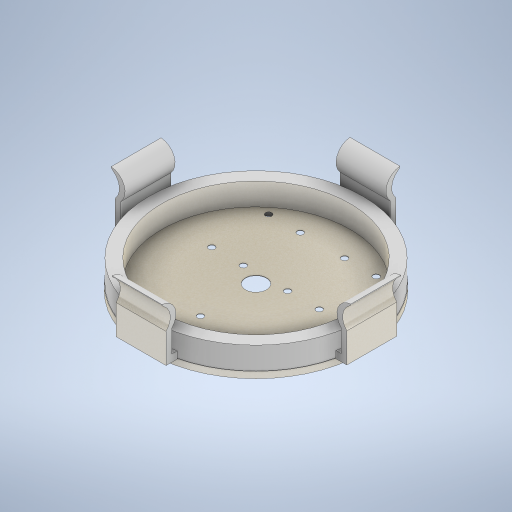
# Autodesk Inventor part: TapaContenedorTest
Saved by Autodesk Inventor 2024 (Build 280153000, 153)
## iProperties
Created: 2024-05-15
Part Number: TapaContenedorTest
Material: Genérico
Document SubType Name: Modeling
Designer: alexa
Density: 1 g/cm^3
Appearance: Valor por defecto
Author: alexa
Autodesk Inventor part; units mm, degrees
ref_plane "YZ Plane" through (0, 0, 0) normal (1, 0, 0) x (0, 1, 0)
ref_plane "XZ Plane" through (0, 0, 0) normal (0, 1, 0) x (-1, 0, 0)
ref_plane "XY Plane" through (0, 0, 0) normal (0, 0, 1) x (1, 0, 0)
sketch "Sketch1" plane through (0, 0, 0) normal (0, 1, 0) x (-1, 0, 0)
  circle A0 centre (0, 0) radius 50.9
  dimension "d0" = 101.8
  constraints: 1 centre point, 1 coincident
  measures "d0" diameter of A0
extrude "Extrusion1" add sketch "Sketch1" along normal blind 0.2
sketch "Sketch2" plane through (0, 0.2, 0) normal (0, 1, 0) x (1, 0, 0)
  circle A0 centre (0, 0) radius 50.675
  circle A1 centre (0, 0) radius 44.675
  dimension "d3" = 6
  dimension "d49" = 89.35
  constraints: 2 centre point, 1 coincident
  measures "d3" radial gap between concentric circles of A0 A1
  measures "d49" diameter of A1
extrude "Extrusion2" add sketch "Sketch2" along normal blind 10.6
sketch "Sketch3" plane through (0, 0, 0) normal (0, -1, 0) x (1, 0, 0)
  circle A0 centre (0, 0) radius 50.9 projected
  line L0 (-54.6995, -11.6386) -> (-54.6995, 12.0614)
  line L1 (-54.6995, -11.6386) -> (-49.5515, -11.6386)
  line L2 (-54.6995, 12.0614) -> (-49.4503, 12.0614)
  dimension "d8" = 23.7
  constraints: 6 end point, 2 point on circle, 1 horizontal, 1 parallel
  measures "d8" distance of L0.start L0.end
extrude "Extrusion3" add sketch "Sketch3" against normal blind 3.4 contours A0 L1 L0 L2
sketch "Sketch4" plane through (0, 3.4, 0) normal (0, 1, 0) x (1, 0, 0)
  line L0 (-54.6995, 11.6386) -> (-54.6995, -12.0614) projected
  line L1 (-54.6995, -12.0614) -> (-51.9995, -12.0614)
  line L2 (-51.9995, -12.0614) -> (-51.9995, 11.6386)
  line L3 (-51.9995, 11.6386) -> (-54.6995, 11.6386)
  line L4 (-54.6995, 11.6386) -> (-54.6995, -12.0614)
  point P0 (0, 0)
  dimension "d11" = 2.7
  constraints: 8 end point, 2 parallel, 1 horizontal, 1 perpendicular
  measures "d11" distance of L3.end L2.end
extrude "Extrusion4" add sketch "Sketch4" along normal blind 10.6
sketch "Sketch6" plane through (-54.6995, 0, 12.0614) normal (0, 0, 1) x (1, 0, 0)
  line L0 (2.7, 14) -> (0, 14) projected
  line L1 (-1.9318, 26) -> (-2.8707, 26)
  arc A0 (2.7, 14) -> (-2.8707, 26) centre (-2.4013, 18.9249) ccw
  arc A1 (0, 14) -> (-5.5707, 26) centre (-5.1013, 18.9249) ccw
  line L2 (-2.8707, 26) -> (-5.5707, 26)
  point P0 (54.6995, 0)
  point P1 (-4.6318, 26)
  point P2 (-4.6318, 26)
  dimension "d15" = 2.7
  dimension "d18" = 2.7
  constraints: 6 point on circle, 4 end point, 3 horizontal, 2 centre point, 5 other
  measures "d15" distance of L0.start L0.end
  measures "d18" distance of A0.centre A1.centre
extrude "Extrusion5" add sketch "Sketch6" against normal blind 23.7 contours L0 A1 L2 L1 A0
fillet "Fillet1" radius 2 1 edges at (-59.3314, 26, 0.2114)
pattern_circular "Circular Pattern1" count 4 over 360 about axis through (0, -10, 0) along (0, 1, 0) of "Fillet1", "Extrusion5", "Extrusion4", "Extrusion3"
sketch "Sketch7" plane through (0, 0.2, 0) normal (0, 1, 0) x (1, 0, 0)
  circle A0 centre (0, 0) radius 5
  dimension "d29" = 10
  constraints: 1 centre point, 1 coincident
  measures "d29" diameter of A0
extrude "Extrusion6" cut sketch "Sketch7" against normal blind 1
sketch "Sketch12" plane through (0, 0, 0) normal (0, -1, 0) x (1, 0, 0)
  circle A0 centre (0.1066, 26.4372) radius 1.5
  circle A1 centre (0.1066, 38.9372) radius 1.5
  line L0 (12.0614, 56.6314) -> (-11.6386, 56.6314) projected
  point P0 (0, 0)
  point P1 (0.2114, 56.6314)
  dimension "d64" = 3
  dimension "d66" = 3
  dimension "d80" = 17.6942
  dimension "d81" = 12.5
  constraints: 2 centre point, 1 midpoint
  measures "d64" diameter of A0
  measures "d66" diameter of A1
  measures "d80" vertical distance of point (0.211, 56.631) A1.centre
  measures "d81" distance of A1.centre A0.centre
extrude "Extrusion11" cut sketch "Sketch12" against normal blind 1
sketch "Sketch13" plane through (0, 0, 0) normal (0, -1, 0) x (1, 0, 0)
  circle A0 centre (10.5, -4.5) radius 1.5
  point P0 (0, 0)
  dimension "d71" = 3
  constraints: 1 centre point
  measures "d71" diameter of A0
extrude "Extrusion12" cut sketch "Sketch13" against normal blind 1
pattern_linear "Rectangular Pattern3" count 2 spacing 15 along (1, 0, 0) count 2 spacing 27 along (0, 0, -1) of "Extrusion12"
mirror "Mirror2" about plane through (0, 0, 0) normal (1, 0, 0) of "Extrusion12", "Rectangular Pattern3"
sketch "Sketch14" plane through (0, 0, 0) normal (0, -1, 0) x (1, 0, 0)
  circle A0 centre (0, 0) radius 50.9
  circle A1 centre (0, 0) radius 43.8
  dimension "d82" = 7.1
  dimension "d83" = 101.8
  constraints: 2 centre point, 2 coincident
  measures "d82" radial gap between concentric circles of A1 A0
  measures "d83" diameter of A0
extrude "Extrusion13" add sketch "Sketch14" along normal blind 2.8
body "Solid1"
